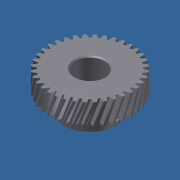
# Autodesk Inventor part: ENGR.HELICOIDAL MOVIDA(59)
Saved by Autodesk Inventor 2012 SP1 (Build 160190100, 190)
## iProperties
Created: 2012-07-24
Part Number: ENGR.HELICOIDAL MOVIDA(59)
Material: Carbon Steel
Document SubType Name: Modeling
Designer: bruno.silveira
Mass: 178.015 g
Surface Area: 47.7522 cm^2
Volume: 22.6195 cm^3
Density: 7.87 g/cm^3
Author: bruno.silveira
Autodesk Inventor part; units mm, degrees
ref_plane "YZ Plane" through (0, 0, 0) normal (1, 0, 0) x (0, 1, 0)
ref_plane "XZ Plane" through (0, 0, 0) normal (0, 1, 0) x (-1, 0, 0)
ref_plane "XY Plane" through (0, 0, 0) normal (0, 0, 1) x (1, 0, 0)
sketch "Sketch1" plane through (0, 0, 0) normal (0, 0, 1) x (1, 0, 0)
  circle A0 centre (0, 0) radius 20
  dimension "d0" = 40
  constraints: 1 centre point, 1 coincident
  measures "d0" diameter of A0
extrude "Extrusion1" add sketch "Sketch1" along normal blind 18
sketch "Sketch2" plane through (0, 0, 0) normal (0, 0, -1) x (-1, 0, 0)
  circle A0 centre (0, 0) radius 20 projected
  circle A1 centre (0, 0) radius 12.5
  dimension "d3" = 25
  constraints: 1 centre point, 1 coincident
  measures "d3" diameter of A1
extrude "Extrusion2" cut sketch "Sketch2" against normal blind 8
spur gear teeth "Spur Gear1" teeth 36 pitch diameter 38.3104 tip diameter 40.3101 root diameter 35.8104 face width 10 helix angle 20 hand right trims to tip circle yes start plane through (0, 0, 18) normal (0, 0, 1) x (1, 0, 0)
sketch "Sketch3" plane through (0, 0, 0) normal (0, 0, -1) x (-1, 0, 0)
  circle A0 centre (0, 0) radius 12.5 projected
  circle A1 centre (0, 0) radius 7
  dimension "d6" = 14
  constraints: 1 centre point, 1 coincident
  measures "d6" diameter of A1
extrude "Extrusion3" cut sketch "Sketch3" against normal blind 20 contours A1
sketch "Sketch4" plane through (0, 0, 0) normal (1, 0, 0) x (0, 1, 0)
  circle A0 centre (0, 4) radius 2
  line L0 (-12.5, 0) -> (12.5, 0) projected
  point P0 (0, 0)
  dimension "d9" = 4
  dimension "d10" = 4
  constraints: 1 centre point
  measures "d9" diameter of A0
  measures "d10" distance from line of L0 A0.centre
extrude "Extrusion4" cut sketch "Sketch4" along normal mid plane 30
fillet "Fillet1" radius 0.5 1 edges at (12.5, 0, 8)
chamfer "Chamfer1" distance 0.5 angle 45 1 edges at (12.5, 0, 0)
chamfer "Chamfer2" distance 0.5 angle 45 2 edges at (7, 0, 0) (7, 0, 18)
body "Solid1"
